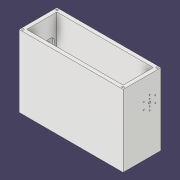
# Autodesk Inventor part: HA005
Saved by Autodesk Inventor 2017 SP1 (Build 210196100, 196)
## iProperties
Created: 2017-06-10
Part Number: HA005
Material: ABS Plastic
Document SubType Name: Modeling
Designer: Zach
Density: 1.06 g/cm^3
Appearance: CR White
Author: Zach
Autodesk Inventor part; units mm, degrees
ref_plane "YZ Plane" through (0, 0, 0) normal (1, 0, 0) x (0, 1, 0)
ref_plane "XZ Plane" through (0, 0, 0) normal (0, 1, 0) x (-1, 0, 0)
ref_plane "XY Plane" through (0, 0, 0) normal (0, 0, 1) x (1, 0, 0)
sketch "Sketch1" plane through (0, 0, 0) normal (0, 0, 1) x (1, 0, 0)
  line L0 (0, 0) -> (275, 0)
  line L1 (275, 0) -> (275, 200)
  line L2 (275, 200) -> (0, 200)
  line L3 (0, 200) -> (0, 0)
  dimension "d0" = 275
  dimension "d1" = 200
  constraints: 8 end point, 2 parallel, 1 horizontal, 1 perpendicular
  measures "d0" distance of L2.end L1.end
  measures "d1" distance of L1.end L0.end
extrude "Extrusion1" add sketch "Sketch1" along normal blind 20
sketch "Sketch3" plane through (0, 0, 20) normal (0, 0, 1) x (1, 0, 0)
  line L0 (275, 0) -> (275, 200) projected
  line L1 (0, 200) -> (275, 200)
  line L2 (275, 200) -> (275, 0)
  line L3 (275, 0) -> (0, 0)
  line L4 (0, 0) -> (0, 200)
  point P0 (0, 0)
  constraints: 8 end point, 2 parallel, 1 coincident, 1 horizontal, 1 perpendicular
extrude "Extrusion3" add sketch "Sketch3" along normal blind 80
sketch "Sketch4" plane through (0, 0, 0) normal (0, -1, 0) x (1, 0, 0)
  circle A0 centre (37.5, 50) radius 17.5 construction
  circle A1 centre (237.5, 50) radius 17.5 construction
  line L0 (37.5, 50) -> (237.5, 50) construction
  line L1 (0, 0) -> (0, 100) projected
  line L2 (0, 100) -> (275, 100) projected
  circle A2 centre (42.5, 55) radius 22.5
  point P0 (0, 50)
  point P1 (137.5, 50)
  point P2 (137.5, 100)
  dimension "d10" = 35
  dimension "d11" = 35
  dimension "d12" = 200
  dimension "d79" = 45
  dimension "d80" = 5
  dimension "d81" = 5
  constraints: 3 centre point, 3 midpoint, 2 end point, 1 horizontal, 1 horizontal alignment, 1 vertical alignment
  measures "d10" diameter of A0
  measures "d11" diameter of A1
  measures "d12" distance of L0.end L0.start
  measures "d79" diameter of A2
  measures "d80" horizontal distance of L0.start A2.centre
  measures "d81" horizontal distance of L0.start A2.centre
extrude "Extrusion4" cut sketch "Sketch4" against normal blind 100
sketch "Sketch5" plane through (0, 200, 0) normal (0, 1, 0) x (1, 0, 0)
  line L0 (275, 0) -> (0, 0) projected
  line L1 (0, 0) -> (0, -100) projected
  line L2 (275, -100) -> (0, -100) projected
  line L3 (275, 0) -> (275, -100) projected
  line L4 (265, -90) -> (10, -90)
  line L5 (10, -90) -> (10, -10)
  line L6 (10, -10) -> (265, -10)
  line L7 (265, -10) -> (265, -90)
  point P0 (0, 0)
  dimension "d15" = 10
  constraints: 8 end point, 3 other
  measures "d15" distance between parallel lines of L3 L7
extrude "Extrusion5" cut sketch "Sketch5" against normal blind 190 contours L4 L5 L6 L7
sketch "Sketch6" plane through (0, 0, 0) normal (-1, 0, 0) x (0, 0, 1)
  line L0 (0, 200) -> (100, 200) projected
  line L1 (0, 200) -> (0, 0) projected
  line L2 (100, 200) -> (0, 200)
  line L3 (0, 200) -> (0, 190)
  line L4 (0, 190) -> (100, 190)
  line L5 (100, 190) -> (100, 200)
  dimension "d18" = 10
  constraints: 8 end point, 2 parallel, 1 horizontal, 1 perpendicular, 1 point on line
  measures "d18" distance of L3.end L2.end
extrude "Extrusion6" cut sketch "Sketch6" against normal through all
sketch "Sketch7" plane through (0, 190, 100) normal (0, 1, 0) x (1, 0, 0)
  line L0 (275, 100) -> (275, 0) construction
  line L1 (0, 100) -> (275, 100) construction
  line L2 (0, 0) -> (0, 100) construction
  line L3 (275, 0) -> (0, 0) construction
  line L4 (265, 10) -> (265, 90) construction
  line L5 (10, 10) -> (265, 10) construction
  line L6 (10, 90) -> (10, 10) construction
  line L7 (265, 90) -> (10, 90) construction
  line L8 (270, 5) -> (270, 95) construction
  line L9 (270, 95) -> (5, 95) construction
  line L10 (5, 95) -> (5, 5) construction
  line L11 (5, 5) -> (270, 5) construction
  circle A0 centre (270, 5) radius 2.5
  circle A1 centre (270, 95) radius 2.5
  circle A2 centre (5, 95) radius 2.5
  circle A3 centre (5, 5) radius 2.5
  point P0 (0, 100)
  dimension "d21" = 5
  dimension "d22" = 5
  dimension "d23" = 5
  dimension "d24" = 5
  dimension "d25" = 5
  constraints: 8 end point, 4 centre point, 4 coincident, 3 other
  measures "d21" distance between parallel lines of L0 L8
  measures "d22" diameter of A0
  measures "d23" diameter of A1
  measures "d24" diameter of A2
  measures "d25" diameter of A3
extrude "Extrusion7" cut sketch "Sketch7" against normal blind 25
sketch "Sketch8" plane through (0, 0, 0) normal (0, -1, 0) x (1, 0, 0)
  line L0 (82, 15) -> (85, 15)
  line L1 (85, 15) -> (85, 30)
  line L2 (85, 30) -> (82, 30)
  line L3 (82, 30) -> (82, 15)
  line L4 (0, 0) -> (0, 100) projected
  line L5 (0, 0) -> (275, 0) projected
  line L6 (97, 15) -> (97, 30)
  line L7 (97, 30) -> (94, 30)
  line L8 (94, 30) -> (94, 15)
  line L9 (94, 15) -> (97, 15)
  line L10 (109, 15) -> (109, 30)
  line L11 (109, 30) -> (106, 30)
  line L12 (106, 30) -> (106, 15)
  line L13 (106, 15) -> (109, 15)
  line L14 (121, 15) -> (121, 30)
  line L15 (121, 30) -> (118, 30)
  line L16 (118, 30) -> (118, 15)
  line L17 (118, 15) -> (121, 15)
  line L18 (133, 15) -> (133, 30)
  line L19 (133, 30) -> (130, 30)
  line L20 (130, 30) -> (130, 15)
  line L21 (130, 15) -> (133, 15)
  line L22 (145, 15) -> (145, 30)
  line L23 (145, 30) -> (142, 30)
  line L24 (142, 30) -> (142, 15)
  line L25 (142, 15) -> (145, 15)
  line L26 (157, 15) -> (157, 30)
  line L27 (157, 30) -> (154, 30)
  line L28 (154, 30) -> (154, 15)
  line L29 (154, 15) -> (157, 15)
  line L30 (169, 15) -> (169, 30)
  line L31 (169, 30) -> (166, 30)
  line L32 (166, 30) -> (166, 15)
  line L33 (166, 15) -> (169, 15)
  line L34 (181, 15) -> (181, 30)
  line L35 (181, 30) -> (178, 30)
  line L36 (178, 30) -> (178, 15)
  line L37 (178, 15) -> (181, 15)
  line L38 (193, 15) -> (193, 30)
  line L39 (193, 30) -> (190, 30)
  line L40 (190, 30) -> (190, 15)
  line L41 (190, 15) -> (193, 15)
  line L42 (205, 15) -> (205, 30)
  line L43 (205, 30) -> (202, 30)
  line L44 (202, 30) -> (202, 15)
  line L45 (202, 15) -> (205, 15)
  line L46 (217, 15) -> (217, 30)
  line L47 (217, 30) -> (214, 30)
  line L48 (214, 30) -> (214, 15)
  line L49 (214, 15) -> (217, 15)
  line L50 (229, 15) -> (229, 30)
  line L51 (229, 30) -> (226, 30)
  line L52 (226, 30) -> (226, 15)
  line L53 (226, 15) -> (229, 15)
  line L54 (241, 15) -> (241, 30)
  line L55 (241, 30) -> (238, 30)
  line L56 (238, 30) -> (238, 15)
  line L57 (238, 15) -> (241, 15)
  dimension "d28" = 3
  dimension "d29" = 15
  dimension "d30" = 82
  dimension "d31" = 15
  dimension "d34" = 12
  constraints: 112 end point, 2 horizontal, 2 parallel, 1 perpendicular, 104 other
  measures "d28" distance of L2.end L1.end
  measures "d29" distance of L1.end L0.end
  measures "d30" distance between parallel lines of L4 L3
  measures "d31" distance between parallel lines of L5 L0
  measures "d34" distance of L0.end L6.start
extrude "Extrusion8" cut sketch "Sketch8" against normal through all contours L3 L2 L1 L0 | L9 L8 L7 L6 | L13 L12 L11 L10 | L17 L16 L15 L14 | L21 L20 L19 L18 | L25 L24 L23 L22 | L29 L28 L27 L26 | L33 L32 L31 L30 | L37 L36 L35 L34 | L41 L40 L39 L38 | L45 L44 L43 L42 | L49 L48 L47 L46 | L53 L52 L51 L50
sketch "Sketch2" plane through (275, 0, 100) normal (1, 0, 0) x (0, 0, -1)
  circle A0 centre (70, 125) radius 3
  line L0 (100, 0) -> (0, 0) projected
  line L1 (100, 0) -> (100, 190) projected
  dimension "d4" = 6
  dimension "d45" = 125
  dimension "d46" = 30
  constraints: 1 centre point
  measures "d4" diameter of A0
  measures "d45" distance from line of A0.centre L0
  measures "d46" distance from line of L1 A0.centre
extrude "Extrusion2" cut sketch "Sketch2" against normal through all
sketch "Sketch11" plane through (10, 10, 90) normal (1, 0, 0) x (0, 0, -1)
  circle A0 centre (60, 123.75) radius 1.5
  circle A1 centre (60, 106.25) radius 1.5
  circle A2 centre (60, 115) radius 3 projected
  line L0 (60, 106.25) -> (60, 123.75) construction
  point P0 (90, -10)
  dimension "d49" = 3
  dimension "d50" = 3
  dimension "d51" = 17.5
  constraints: 2 centre point, 2 end point, 1 coincident, 1 midpoint, 1 vertical
  measures "d49" diameter of A0
  measures "d50" diameter of A1
  measures "d51" distance of L0.start L0.end
extrude "Extrusion11" cut sketch "Sketch11" along normal through all both and the other way through all contours A0 | A1
sketch "Sketch12" plane through (10, 10, 90) normal (1, 0, 0) x (0, 0, -1)
  circle A0 centre (60, 115) radius 3 projected
  circle A1 centre (60, 115) radius 5
  point P0 (90, -10)
  dimension "d54" = 10
  constraints: 1 centre point, 1 coincident
  measures "d54" diameter of A1
extrude "Extrusion12" cut sketch "Sketch12" against normal blind 8
sketch "Sketch13" plane through (10, 10, 90) normal (1, 0, 0) x (0, 0, -1)
  circle A0 centre (60, 115) radius 5 projected
  circle A1 centre (60, 115) radius 3 projected
  circle A2 centre (60, 115) radius 14
  point P0 (90, -10)
  dimension "d57" = 28
  constraints: 1 centre point, 1 coincident
  measures "d57" diameter of A2
extrude "Extrusion13" cut sketch "Sketch13" against normal blind 5 contours A2
sketch "Sketch15" plane through (265, 10, 10) normal (-1, 0, 0) x (0, 0, 1)
  circle A0 centre (20, 115) radius 14 projected
  point P0 (-10, -10)
extrude "Extrusion15" cut sketch "Sketch15" against normal blind 5
sketch "Sketch16" plane through (275, 0, 100) normal (1, 0, 0) x (0, 0, -1)
  circle A0 centre (70, 125) radius 3 projected
  circle A1 centre (70, 143) radius 1.5
  circle A2 centre (54.4115, 134) radius 1.5
  circle A3 centre (54.4115, 116) radius 1.5
  circle A4 centre (70, 107) radius 1.5
  circle A5 centre (85.5885, 116) radius 1.5
  circle A6 centre (85.5885, 134) radius 1.5
  point P0 (100, 0)
  dimension "d65" = 3
  dimension "d66" = 18
  dimension "d69" = 360
  constraints: 6 centre point, 1 vertical alignment, 13 other
  measures "d65" diameter of A1
  measures "d66" distance of A0.centre A1.centre
extrude "Extrusion16" cut sketch "Sketch16" against normal blind 10
sketch "Sketch17" plane through (0, 0, 0) normal (0, -1, 0) x (1, 0, 0)
  line L0 (82, 65) -> (229, 65)
  line L1 (229, 65) -> (229, 45)
  line L2 (229, 45) -> (82, 45)
  line L3 (82, 45) -> (82, 65)
  circle A0 centre (42.5, 55) radius 22.5 projected
  line L4 (10, 10) -> (265, 10) projected
  line L5 (229, 45) -> (229, 65)
  line L6 (229, 30) -> (229, 15) projected
  line L7 (82, 15) -> (82, 30) projected
  point P0 (137.5, 10)
  point P1 (82, 55)
  point P2 (137.5, 10)
  point P3 (229, 22.5)
  point P4 (229, 22.5)
  point P5 (82, 22.5)
  dimension "d93" = 20
  constraints: 10 end point, 5 midpoint, 2 parallel, 2 vertical alignment, 1 horizontal, 1 horizontal alignment, 1 perpendicular
  measures "d93" distance of L0.end L1.end
extrude "Extrusion17" [suppressed]
sketch "Sketch18" plane through (10, 10, 90) normal (1, 0, 0) x (0, 0, -1)
  circle A0 centre (60, 115) radius 14 construction
  line L0 (80, 180) -> (0, 180) construction
  line L1 (0, 180) -> (0, 0) construction
  line L2 (0, 0) -> (80, 0) construction
  line L3 (80, 180) -> (80, 0) construction
  line L4 (80, 0) -> (70.0241, 84.4126)
  line L5 (70.0241, 84.4126) -> (80, 84.4126)
  line L6 (80, 0) -> (80, 84.4126)
  line L7 (70.0241, 84.4126) -> (80, 110)
  line L8 (80, 84.4126) -> (80, 110)
  point P0 (90, -10)
  dimension "d82" = 6.74
  dimension "d84" = 85
  dimension "d85" = 5
  constraints: 10 end point, 2 collinear, 2 point on line, 1 perpendicular
  measures "d82" angle of L3 L4
  measures "d84" distance of L2.end L4.end
  measures "d85" vertical distance of A0.centre L7.end
extrude "Extrusion18" [suppressed]
fillet "Fillet2" [suppressed]
sketch "Sketch19" plane through (0, 0, 0) normal (0, -1, 0) x (1, 0, 0)
  line L0 (82, 65) -> (229, 65) construction
  line L1 (82, 65) -> (42.5, 65)
  line L2 (42.5, 65) -> (42.5, 45)
  line L3 (42.5, 45) -> (82, 45)
  line L4 (82, 45) -> (82, 65)
  circle A0 centre (42.5, 55) radius 22.5 construction
  point P0 (0, 0)
  constraints: 8 end point, 2 coincident, 2 parallel, 1 horizontal, 1 midpoint, 1 perpendicular
extrude "Extrusion19" [suppressed]
sketch "Sketch20" plane through (0, 0, 0) normal (0, -1, 0) x (1, 0, 0)
  circle A0 centre (92.5, 55) radius 20
  arc A1 (65, 55) -> (65, 55) centre (42.5, 55) ccw projected
  point P0 (0, 0)
  dimension "d97" = 40
  dimension "d98" = 50
  constraints: 1 centre point, 1 horizontal alignment
  measures "d97" diameter of A0
  measures "d98" distance of A0.centre A1.centre
extrude "Extrusion20" [suppressed]
chamfer "Chamfer2" [suppressed]
sketch "Sketch21" plane through (0, 0, 0) normal (0, -1, 0) x (1, 0, 0)
  line L0 (217, 30) -> (217, 15) projected
  line L1 (217, 15) -> (214, 15) projected
  line L2 (214, 15) -> (214, 30) projected
  line L3 (214, 30) -> (217, 30) projected
  line L4 (193, 30) -> (193, 15) projected
  line L5 (193, 15) -> (190, 15) projected
  line L6 (190, 15) -> (190, 30) projected
  line L7 (190, 30) -> (193, 30) projected
  line L8 (169, 30) -> (169, 15) projected
  line L9 (169, 15) -> (166, 15) projected
  line L10 (166, 15) -> (166, 30) projected
  line L11 (166, 30) -> (169, 30) projected
  line L12 (145, 30) -> (145, 15) projected
  line L13 (145, 15) -> (142, 15) projected
  line L14 (142, 15) -> (142, 30) projected
  line L15 (142, 30) -> (145, 30) projected
  line L16 (121, 30) -> (121, 15) projected
  line L17 (121, 15) -> (118, 15) projected
  line L18 (118, 15) -> (118, 30) projected
  line L19 (118, 30) -> (121, 30) projected
  line L20 (97, 30) -> (97, 15) projected
  line L21 (97, 15) -> (94, 15) projected
  line L22 (94, 15) -> (94, 30) projected
  line L23 (94, 30) -> (97, 30) projected
  line L24 (85, 30) -> (85, 15) projected
  line L25 (85, 15) -> (82, 15) projected
  line L26 (82, 15) -> (82, 30) projected
  line L27 (82, 30) -> (85, 30) projected
  line L28 (109, 30) -> (109, 15) projected
  line L29 (109, 15) -> (106, 15) projected
  line L30 (106, 15) -> (106, 30) projected
  line L31 (106, 30) -> (109, 30) projected
  line L32 (133, 30) -> (133, 15) projected
  line L33 (133, 15) -> (130, 15) projected
  line L34 (130, 15) -> (130, 30) projected
  line L35 (130, 30) -> (133, 30) projected
  line L36 (157, 30) -> (157, 15) projected
  line L37 (157, 15) -> (154, 15) projected
  line L38 (154, 15) -> (154, 30) projected
  line L39 (154, 30) -> (157, 30) projected
  line L40 (181, 30) -> (181, 15) projected
  line L41 (181, 15) -> (178, 15) projected
  line L42 (178, 15) -> (178, 30) projected
  line L43 (178, 30) -> (181, 30) projected
  line L44 (205, 30) -> (205, 15) projected
  line L45 (205, 15) -> (202, 15) projected
  line L46 (202, 15) -> (202, 30) projected
  line L47 (202, 30) -> (205, 30) projected
  line L48 (229, 30) -> (229, 15) projected
  line L49 (229, 15) -> (226, 15) projected
  line L50 (226, 15) -> (226, 30) projected
  line L51 (226, 30) -> (229, 30) projected
  circle A0 centre (42.5, 55) radius 22.5 projected
  line L52 (0, 0) -> (275, 0) projected
  line L53 (275, 0) -> (275, 100) projected
  line L54 (0, 100) -> (275, 100) construction
  line L55 (0, 0) -> (0, 100) projected
extrude "Extrusion21" add sketch "Sketch21" against normal blind 10
sketch "Sketch22" plane through (0, 0, 0) normal (0, -1, 0) x (1, 0, 0)
  line L0 (80.7735, 55) -> (69.2265, 55)
  line L1 (69.2265, 55) -> (63.453, 65)
  line L2 (63.453, 65) -> (69.2265, 75)
  line L3 (69.2265, 75) -> (80.7735, 75)
  line L4 (80.7735, 75) -> (86.547, 65)
  line L5 (86.547, 65) -> (80.7735, 55)
  line L6 (211.547, 65) -> (205.7735, 55)
  line L7 (205.7735, 55) -> (194.2265, 55)
  line L8 (194.2265, 55) -> (188.453, 65)
  line L9 (188.453, 65) -> (194.2265, 75)
  line L10 (194.2265, 75) -> (205.7735, 75)
  line L11 (205.7735, 75) -> (211.547, 65)
  line L12 (75, 65) -> (200, 65) construction
  line L13 (0, 100) -> (275, 100) projected
  line L14 (80.7735, 75) -> (194.2265, 75)
  line L15 (194.2265, 55) -> (80.7735, 55)
  point P0 (0, 0)
  point P1 (137.5, 65)
  point P2 (137.5, 100)
  dimension "d106" = 20
  dimension "d107" = 20
  dimension "d108" = 125
  dimension "d109" = 35
  constraints: 30 end point, 3 horizontal alignment, 2 midpoint, 1 horizontal, 1 vertical alignment, 26 other
  measures "d106" distance between parallel lines of L0 L3
  measures "d107" distance between parallel lines of L7 L10
  measures "d108" distance of L12.start L12.end
  measures "d109" distance between parallel lines of L13 L12
extrude "Extrusion22" cut sketch "Sketch22" against normal blind 10
sketch "Sketch24" plane through (0, 0, 0) normal (0, -1, 0) x (1, 0, 0)
  line L0 (235, 35) -> (232, 35)
  line L1 (232, 35) -> (232, 20)
  line L2 (232, 20) -> (235, 20)
  line L3 (235, 20) -> (235, 35)
  line L4 (10, 10) -> (265, 10) projected
  line L5 (275, 0) -> (275, 100) projected
  line L6 (227, 35) -> (224, 35)
  line L7 (224, 35) -> (224, 20)
  line L8 (224, 20) -> (227, 20)
  line L9 (227, 20) -> (227, 35)
  line L10 (219, 35) -> (216, 35)
  line L11 (216, 35) -> (216, 20)
  line L12 (216, 20) -> (219, 20)
  line L13 (219, 20) -> (219, 35)
  line L14 (211, 35) -> (208, 35)
  line L15 (208, 35) -> (208, 20)
  line L16 (208, 20) -> (211, 20)
  line L17 (211, 20) -> (211, 35)
  line L18 (203, 35) -> (200, 35)
  line L19 (200, 35) -> (200, 20)
  line L20 (200, 20) -> (203, 20)
  line L21 (203, 20) -> (203, 35)
  line L22 (195, 35) -> (192, 35)
  line L23 (192, 35) -> (192, 20)
  line L24 (192, 20) -> (195, 20)
  line L25 (195, 20) -> (195, 35)
  line L26 (187, 35) -> (184, 35)
  line L27 (184, 35) -> (184, 20)
  line L28 (184, 20) -> (187, 20)
  line L29 (187, 20) -> (187, 35)
  line L30 (179, 35) -> (176, 35)
  line L31 (176, 35) -> (176, 20)
  line L32 (176, 20) -> (179, 20)
  line L33 (179, 20) -> (179, 35)
  line L34 (171, 35) -> (168, 35)
  line L35 (168, 35) -> (168, 20)
  line L36 (168, 20) -> (171, 20)
  line L37 (171, 20) -> (171, 35)
  line L38 (163, 35) -> (160, 35)
  line L39 (160, 35) -> (160, 20)
  line L40 (160, 20) -> (163, 20)
  line L41 (163, 20) -> (163, 35)
  line L42 (155, 35) -> (152, 35)
  line L43 (152, 35) -> (152, 20)
  line L44 (152, 20) -> (155, 20)
  line L45 (155, 20) -> (155, 35)
  line L46 (147, 35) -> (144, 35)
  line L47 (144, 35) -> (144, 20)
  line L48 (144, 20) -> (147, 20)
  line L49 (147, 20) -> (147, 35)
  line L50 (139, 35) -> (136, 35)
  line L51 (136, 35) -> (136, 20)
  line L52 (136, 20) -> (139, 20)
  line L53 (139, 20) -> (139, 35)
  line L54 (131, 35) -> (128, 35)
  line L55 (128, 35) -> (128, 20)
  line L56 (128, 20) -> (131, 20)
  line L57 (131, 20) -> (131, 35)
  line L58 (123, 35) -> (120, 35)
  line L59 (120, 35) -> (120, 20)
  line L60 (120, 20) -> (123, 20)
  line L61 (123, 20) -> (123, 35)
  line L62 (115, 35) -> (112, 35)
  line L63 (112, 35) -> (112, 20)
  line L64 (112, 20) -> (115, 20)
  line L65 (115, 20) -> (115, 35)
  line L66 (107, 35) -> (104, 35)
  line L67 (104, 35) -> (104, 20)
  line L68 (104, 20) -> (107, 20)
  line L69 (107, 20) -> (107, 35)
  line L70 (99, 35) -> (96, 35)
  line L71 (96, 35) -> (96, 20)
  line L72 (96, 20) -> (99, 20)
  line L73 (99, 20) -> (99, 35)
  line L74 (91, 35) -> (88, 35)
  line L75 (88, 35) -> (88, 20)
  line L76 (88, 20) -> (91, 20)
  line L77 (91, 20) -> (91, 35)
  line L78 (83, 35) -> (80, 35)
  line L79 (80, 35) -> (80, 20)
  line L80 (80, 20) -> (83, 20)
  line L81 (83, 20) -> (83, 35)
  line L82 (75, 35) -> (72, 35)
  line L83 (72, 35) -> (72, 20)
  line L84 (72, 20) -> (75, 20)
  line L85 (75, 20) -> (75, 35)
  line L86 (67, 35) -> (64, 35)
  line L87 (64, 35) -> (64, 20)
  line L88 (64, 20) -> (67, 20)
  line L89 (67, 20) -> (67, 35)
  line L90 (59, 35) -> (56, 35)
  line L91 (56, 35) -> (56, 20)
  line L92 (56, 20) -> (59, 20)
  line L93 (59, 20) -> (59, 35)
  line L94 (51, 35) -> (48, 35)
  line L95 (48, 35) -> (48, 20)
  line L96 (48, 20) -> (51, 20)
  line L97 (51, 20) -> (51, 35)
  line L98 (43, 35) -> (40, 35)
  line L99 (40, 35) -> (40, 20)
  line L100 (40, 20) -> (43, 20)
  line L101 (43, 20) -> (43, 35)
  line L102 (40, 27.5) -> (235, 27.5)
  point P0 (0, 0)
  point P1 (137.5, 27.5)
  point P2 (137.5, 10)
  dimension "d112" = 3
  dimension "d113" = 15
  dimension "d114" = 10
  dimension "d118" = 8
  constraints: 202 end point, 4 midpoint, 2 horizontal, 2 parallel, 1 perpendicular, 1 vertical alignment, 192 other
  measures "d112" distance of L2.end L1.end
  measures "d113" distance of L1.end L0.end
  measures "d114" distance between parallel lines of L4 L2
  measures "d118" distance of L0.start L6.start
extrude "Extrusion23" cut sketch "Sketch24" against normal blind 10
sketch "Sketch25" plane through (10, 10, 10) normal (0, 0, 1) x (1, 0, 0)
  circle A0 centre (127.5, 15) radius 3
  line L0 (-10, -10) -> (265, -10) projected
  point P0 (127.5, -10)
  dimension "d125" = 6
  dimension "d126" = 25
  constraints: 1 centre point, 1 midpoint, 1 vertical alignment
  measures "d125" diameter of A0
  measures "d126" distance from line of A0.centre L0
extrude "Extrusion24" cut sketch "Sketch25" against normal through all
sketch "Sketch26" plane through (0, 10, 0) normal (0, 1, 0) x (1, 0, 0)
  circle A0 centre (205, -65) radius 16
  circle A1 centre (70, -65) radius 16
  line L0 (205, -65) -> (70, -65) construction
  line L1 (10, -90) -> (265, -90) projected
  line L2 (205, -81) -> (70, -81)
  line L3 (205, -49) -> (70, -49)
  arc A2 (205, -81) -> (205, -49) centre (205, -65) ccw
  arc A3 (70, -49) -> (70, -81) centre (70, -65) ccw
  point P0 (0, 0)
  point P1 (137.5, -65)
  point P2 (137.5, -90)
  point P3 (211.547, -65)
  dimension "d129" = 32
  dimension "d130" = 32
  dimension "d131" = 135
  constraints: 8 point on circle, 7 tangent, 6 end point, 4 centre point, 2 midpoint, 1 horizontal, 1 horizontal alignment, 1 vertical alignment
  measures "d129" diameter of A0
  measures "d130" diameter of A1
  measures "d131" distance of L0.start L0.end
extrude "Extrusion25" cut sketch "Sketch26" against normal blind 8
sketch "Sketch27" plane through (10, 10, 10) normal (0, 0, 1) x (1, 0, 0)
  circle A0 centre (127.5, 15) radius 3 projected
  line L0 (157.5, -8) -> (97.5, -8)
  line L1 (97.5, -8) -> (97.5, 52)
  line L2 (97.5, 52) -> (157.5, 52)
  line L3 (157.5, 52) -> (157.5, -8)
  point P0 (-10, -10)
  point P1 (97.5, 22)
  point P2 (127.5, -8)
  dimension "d134" = 60
  dimension "d135" = 60
  dimension "d138" = 37
  constraints: 8 end point, 2 midpoint, 2 parallel, 1 horizontal, 1 perpendicular, 1 vertical alignment
  measures "d134" distance of L0.end L1.end
  measures "d135" distance of L1.end L2.end
  measures "d138" distance from line of L2 A0.centre
extrude "Extrusion26" add sketch "Sketch27" along normal blind 21
sketch "Sketch28" plane through (10, 10, 31) normal (0, 0, 1) x (1, 0, 0)
  line L0 (60, 0) -> (195, 0) projected
  line L1 (60, 0) -> (60, -8) projected
  line L2 (60, -8) -> (195, -8) projected
  line L3 (195, 0) -> (195, -8) projected
  line L4 (157.5, 52) -> (157.5, 0) projected
  line L5 (157.5, 0) -> (97.5, 0)
  line L6 (97.5, 0) -> (97.5, -8)
  line L7 (97.5, -8) -> (157.5, -8)
  line L8 (157.5, -8) -> (157.5, 0)
  line L9 (97.5, 0) -> (97.5, 52) projected
  point P0 (-10, -10)
  constraints: 8 end point, 2 parallel, 2 point on line, 1 horizontal, 1 perpendicular
extrude "Extrusion27" cut sketch "Sketch28" along normal blind 20 contours L0 L8 L2 L6
sketch "Sketch30" plane through (0, 0, 0) normal (0, 0, -1) x (-1, 0, 0)
  circle A0 centre (-137.5, 25) radius 3 projected
  circle A1 centre (-137.5, 25) radius 3 projected
  circle A2 centre (-137.5, 25) radius 7.5
  point P0 (0, 0)
  dimension "d141" = 15
  constraints: 1 centre point, 1 coincident
  measures "d141" diameter of A2
extrude "Extrusion28" cut sketch "Sketch30" against normal blind 20
chamfer "Chamfer3" distance 2 angle 45 6 edges at (137.5, 0, 75) (66.3397, 0, 60) (66.3397, 0, 70) (137.5, 0, 55) (208.6603, 0, 60) (208.6603, 0, 70)
body "Solid1"
